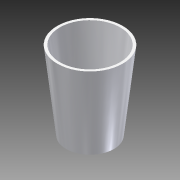
# Autodesk Inventor part: Trash Can Bottom
Saved by Autodesk Inventor 2014 SP2 (Build 180246200, 246)
## iProperties
Created: 2014-09-17
Part Number: Trash Can Bottom
Material: Polypropylene
Document SubType Name: Modeling
Designer: Sophiagirraffe
Density: 0.899 g/cm^3
Appearance: PVC - White
Author: Sophiagirraffe
Autodesk Inventor part; units mm, degrees
ref_plane "YZ Plane" through (0, 0, 0) normal (1, 0, 0) x (0, 1, 0)
ref_plane "XZ Plane" through (0, 0, 0) normal (0, 1, 0) x (-1, 0, 0)
ref_plane "XY Plane" through (0, 0, 0) normal (0, 0, 1) x (1, 0, 0)
sketch "Sketch1" plane through (0, 0, 0) normal (0, 1, 0) x (-1, 0, 0)
  circle A0 centre (0, 0) radius 120.65
  dimension "d0" = 241.3
  constraints: 1 centre point, 1 coincident
  measures "d0" diameter of A0
sketch "Sketch2" plane through (0, 0, 0) normal (0, 1, 0) x (-1, 0, 0)
  circle A0 centre (0, 0) radius 5.5202
  constraints: 1 centre point, 1 coincident
extrude "Extrusion1" add sketch "Sketch2" along normal blind 395.2875
sketch "Sketch3" plane through (0, 395.2875, 0) normal (0, 1, 0) x (1, 0, 0)
  circle A0 centre (0, 0) radius 5.5202 projected
  circle A1 centre (0, 0) radius 165.1
  dimension "d3" = 330.2
  constraints: 1 centre point, 1 coincident
  measures "d3" diameter of A1
loft "Loft1" add profiles "Sketch1", "Sketch3" contours all / A0 | A1
shell "Shell1" thickness 12.7 removed faces 1 at (-20.3699, 395.2875, -51.1247)
body "Solid1"
